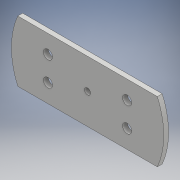
# Autodesk Inventor part: podstawa2
Saved by Autodesk Inventor 2017.3 (Build 213256000, 256)
## iProperties
Created: 2019-03-17
Part Number: podstawa2
Material: Ogólny
Document SubType Name: Modeling
Designer: legox
Density: 1 g/cm^3
Appearance: Domyślna
Author: legox
Autodesk Inventor part; units mm, degrees
ref_plane "YZ Plane" through (0, 0, 0) normal (1, 0, 0) x (0, 1, 0)
ref_plane "XZ Plane" through (0, 0, 0) normal (0, 1, 0) x (-1, 0, 0)
ref_plane "XY Plane" through (0, 0, 0) normal (0, 0, 1) x (1, 0, 0)
sketch "Szkic1" plane through (0, 0, 0) normal (0, 1, 0) x (-1, 0, 0)
  circle A0 centre (0, 0) radius 25
  circle A1 centre (-13, 4) radius 1.5
  circle A2 centre (-13, -4) radius 1.5
  circle A3 centre (13, 4) radius 1.5
  circle A4 centre (13, -4) radius 1.5
  line L0 (22.9129, -10) -> (-22.9129, -10)
  line L1 (22.9129, 10) -> (-22.9129, 10)
  circle A5 centre (0, 0) radius 1
  dimension "d0" = 50
  dimension "d1" = 3
  dimension "d2" = 13
  dimension "d3" = 4
  dimension "d10" = 2
  constraints: 6 centre point, 4 end point, 4 point on circle, 3 coincident, 2 horizontal
  measures "d0" diameter of A0
  measures "d1" diameter of A1
  measures "d2" horizontal distance of A1.centre point (0, 0)
  measures "d3" vertical distance of point (0, 0) A1.centre
  measures "d10" diameter of A5
extrude "Wyciągnięcie proste3" add sketch "Szkic1" along normal blind 1.6 contours A0 L0 L1
